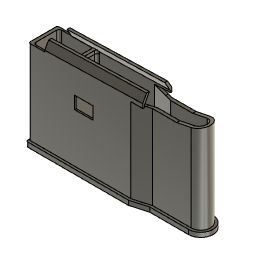
desert_tech_srs_magazine (Autodesk Fusion 360 design; units mm, degrees)
Autodesk Fusion 360 part; units mm, degrees
sketch "Sketch1" plane through (0, 0, 0) normal (0, 0, 1) x (1, 0, 0)
  line L0 (1.5, 0) -> (63.5, 0)
  line L1 (104.5, -3.8188) -> (104.5, 21.8188) construction
  line L2 (63.5, 18) -> (1.5, 18)
  line L3 (0, 16.25) -> (0, 1.5)
  line L4 (63.5, 18) -> (74, 15)
  line L5 (74, 15) -> (98, 15)
  line L6 (0, 9) -> (104.5, 9) construction
  arc A0 (104, 9) -> (98, 15) centre (98, 9) ccw
  line L7 (63.5, 0) -> (74, 3)
  line L8 (74, 3) -> (98, 3)
  arc A1 (98, 3) -> (104, 9) centre (98, 9) ccw
  line L9 (23.5, 15.5) -> (23.5, 10.6624)
  line L10 (25.5, 11.5003) -> (25.5, 15.5)
  line L11 (23.5, 2.5) -> (23.5, 7.3376)
  line L12 (25.5, 6.4997) -> (25.5, 2.5)
  arc A2 (100.0392, 12.4412) -> (98, 13) centre (98, 9) ccw
  line L13 (75.242, 13) -> (98, 13)
  line L14 (61.242, 17) -> (75.242, 13)
  line L15 (2, 15.5) -> (2, 2.5)
  line L16 (61.014, 1) -> (75.014, 5)
  line L17 (75.014, 5) -> (98, 5)
  arc A3 (98, 5) -> (100.0392, 12.4412) centre (98, 9) ccw
  line L18 (61.242, 17) -> (27, 17)
  line L19 (22, 17) -> (3.5, 17)
  line L20 (3.5, 1) -> (22, 1)
  line L21 (27, 1) -> (61.014, 1)
  line L22 (0, 1.5) -> (0, 0)
  line L23 (0, 0) -> (1.5, 0)
  line L24 (0, 16.25) -> (0, 18)
  line L25 (0, 18) -> (1.5, 18)
  line L26 (23.5, 10.6624) -> (23.5, 7.3376)
  line L27 (25.5, 11.5003) -> (25.5, 6.4997)
  arc A4 (27, 17) -> (25.5, 15.5) centre (27, 15.5) ccw
  arc A5 (25.5, 2.5) -> (27, 1) centre (27, 2.5) ccw
  arc A6 (23.5, 15.5) -> (22, 17) centre (22, 15.5) ccw
  arc A7 (22, 1) -> (23.5, 2.5) centre (22, 2.5) ccw
  arc A8 (3.5, 17) -> (2, 15.5) centre (3.5, 15.5) ccw
  arc A9 (2, 2.5) -> (3.5, 1) centre (3.5, 2.5) ccw
  point P0 (0, 18)
  dimension "d2" = 18
  dimension "d3" = 63.5
  dimension "d4" = 24
  dimension "d5" = 6.5
  dimension "d6" = 12
  dimension "d9" = 104.5
  dimension "d21" = 79
  dimension "d23" = 2
  dimension "d40" = 1
  dimension "d41" = 2
  dimension "d42" = 2
  dimension "d59" = 1.5
  dimension "d60" = 1.5
  dimension "d61" = 1.5
  dimension "d62" = 1.5
  dimension "d63" = 1.5
  dimension "d64" = 1.5
  dimension "d65" = 1
  constraint horizontal L0
  constraint vertical L1
  constraint horizontal L2
  constraint vertical L3
  constraint coincident L22.end L23.start
  constraint parallel L2 L5
  constraint midpoint L1 L6.end
  constraint coincident L6 A0.centre
  constraint tangent L5 A0
  constraint coincident L6 A0.start
  constraint symmetric L2.start L6 L0.end
  constraint symmetric L4.end L6 L7.end
  constraint symmetric L5.end L6 L8.end
  constraint symmetric L6 A0 A1
  constraint symmetric L6 A0.start A1.end
  constraint coincident L3 L6.start
  constraint coincident P0 L2
  constraint coincident P0 L3
  constraint coincident L22.end L3
  constraint coincident L22.end L0
  constraint symmetric L0 L2 L6
  constraint vertical L9
  constraint vertical L10
  constraint symmetric L6 L9.end L11.end
  constraint symmetric L6 L10.start L12.start
  constraint concentric A0 A2
  constraint parallel L5 L13
  constraint parallel L4 L14
  constraint parallel L2 L18
  constraint parallel L3 L15
  constraint parallel L0 L20
  constraint parallel L7 L16
  constraint parallel L8 L17
  constraint concentric A1 A3
  constraint tangent A2 A3
  constraint tangent A2 L13
  constraint tangent L17 A3
  constraint collinear L18 L19
  constraint collinear L20 L21
  constraint coincident P0 L24.end
  constraint parallel L12 L27
  constraint tangent L10 A4
  constraint tangent L18 A4
  constraint tangent L12 A5
  constraint tangent L21 A5
  constraint tangent L19 A6
  constraint tangent L9 A6
  constraint tangent L11 A7
  constraint tangent L20 A7
  constraint tangent L15 A8
  constraint tangent L19 A8
  constraint tangent L15 A9
  constraint tangent L20 A9
  constraint vertical L11
  measures "d2" distance of L22.end P0
  measures "d3" distance of L3 L2.start
  measures "d4" distance of L4.end L5.end
  measures "d5" distance of L1 L5.end
  measures "d6" diameter of A0
  measures "d9" distance of L1 L3
  measures "d21" distance of L1 L10
  measures "d23" distance of L9 L10
  measures "d40" distance of L2 L19
  measures "d41" distance of L5 L13
  measures "d42" distance of L3 L15
  measures "d59" radius of A4
  measures "d60" radius of A5
  measures "d61" radius of A6
  measures "d62" radius of A7
  measures "d63" radius of A8
  measures "d64" radius of A9
  measures "d65" distance of L0 L20
extrude "Extrude1" add sketch "Sketch1" along normal blind 55
sketch "Sketch2" plane through (0, 0, 0) normal (0, -1, 0) x (1, 0, 0)
  line L0 (0, 0) -> (63.5, 0)
  line L1 (63.5, 0) -> (63.5, 55)
  line L2 (63.5, 55) -> (0, 55)
  line L3 (28.5, 41) -> (40, 41)
  line L4 (40, 41) -> (40, 33.25)
  line L5 (40, 33.25) -> (28.5, 33.25)
  line L6 (28.5, 33.25) -> (28.5, 41)
  line L7 (0, 55) -> (0, 0)
  line L8 (0, 0) -> (0, 55)
  dimension "d25" = 7.75
  dimension "d26" = 11.5
  dimension "d28" = 14
  dimension "d36" = 28.5
  constraint horizontal L3
  constraint vertical L4
  constraint horizontal L5
  constraint vertical L6
  measures "d25" distance of L3 L5
  measures "d26" distance of L4 L6
  measures "d28" distance of L2 L3
  measures "d36" distance of L6 L8
extrude "Extrude2" cut sketch "Sketch2" against normal up to surface (1 mm away) contours L3 L4 L5 L6
sketch "Sketch4" plane through (0, 0, 0) normal (0, 1, 0) x (1, 0, 0)
  line L0 (0, -60) -> (70.8023, -62) construction
  line L1 (71, -55) -> (0, -55) construction
  line L2 (63.5, 0) -> (63.5, -55)
  line L3 (70.8023, -62) -> (71, -55)
  line L4 (63.5, -55) -> (74, -55)
  line L5 (0, -60) -> (0, -55) construction
  line L6 (10, -55) -> (10, -60.2825)
  line L7 (0, 0) -> (0, -55)
  line L8 (10, -60.2825) -> (70.8023, -62)
  line L9 (10, -55) -> (71, -55)
  point P0 (0, -55)
  dimension "d37" = 7
  dimension "d38" = 7.5
  dimension "d47" = 5
  dimension "d50" = 10
  constraint perpendicular L0 L3
  constraint coincident P0 L1.end
  constraint coincident L1.start L4
  constraint perpendicular L1 L5
  constraint coincident L1 L6.start
  constraint coincident L0 L6.end
  constraint perpendicular L1 L6
  measures "d37" distance of L0.end L1
  measures "d38" distance of L2.end L1.start
  measures "d47" distance of L1 L0.start
  measures "d50" distance of L6 L7
extrude "Extrude3" add sketch "Sketch4" along normal up to surface (18 mm away)
sketch "Sketch5" plane through (72.4958, 0, 2.0478) normal (0.999601, 0, 0.028236) x (0, 1, 0)
  line L0 (18, 52.9733) -> (18, 59.9761)
  line L1 (0, 59.9761) -> (0, 52.9733)
  line L2 (2.1429, 52.9733) -> (3.8531, 52.9733)
  line L3 (9, 63.92) -> (9, 36.6061) construction
  line L4 (1, 54.3074) -> (1, 52.9733)
  line L5 (0, 52.9733) -> (2.2125, 52.9733)
  line L6 (2.2125, 52.9733) -> (12.4801, 52.9733)
  line L7 (12.4801, 52.9733) -> (12.4801, 52.9731)
  line L8 (12.4801, 52.9731) -> (15.5375, 52.9731)
  line L9 (15.5375, 52.9731) -> (12.4801, 52.9731)
  line L10 (17.4429, 59.9761) -> (0, 59.9761)
  line L11 (0, 59.9761) -> (0, 52.9733)
  line L12 (1, 54.3074) -> (4.2, 59.9761)
  line L13 (0, 55.5873) -> (2.4775, 59.9761)
  line L14 (17, 54.3074) -> (13.8, 59.9761)
  line L15 (18, 55.5873) -> (15.5225, 59.9761)
  line L16 (17, 54.3074) -> (17, 52.9733)
  line L17 (18, 59.9761) -> (0, 59.9761)
  line L18 (0, 52.9733) -> (2.1429, 52.9733)
  line L19 (3.8531, 52.9733) -> (14.212, 52.9733)
  line L20 (14.212, 52.9733) -> (15.8571, 52.9733)
  line L21 (15.8571, 52.9733) -> (18, 52.9733)
  line L22 (18, 52.9733) -> (18, 59.9761)
  line L23 (18, 59.9761) -> (17.4429, 59.9761)
  dimension "d49" = 1.5
  dimension "d51" = 1
  dimension "d56" = 9.6
  constraint vertical L3
  constraint symmetric L0 L1 L3
  constraint coincident L10 L12.end
  constraint coincident L11 L13.start
  constraint coincident L10 L13.end
  constraint parallel L12 L13
  constraint parallel L1 L4
  constraint symmetric L3 L4.end L16.end
  constraint symmetric L3 L4.start L14.start
  constraint symmetric L3 L12.end L14.end
  constraint symmetric L3 L13.start L15.start
  constraint symmetric L3 L13.end L15.end
  constraint parallel L2 L6
  constraint parallel L1 L11
  constraint collinear L6 L19
  constraint horizontal L10
  constraint coincident L0.start L21.end
  constraint perpendicular L21 L22
  constraint coincident L15.start L22
  constraint collinear L10 L17
  constraint collinear L10 L23
  measures "d49" distance of L12 L13
  measures "d51" distance of L4 L11
  measures "d56" distance of L12.end L14.end
extrude "Extrude4" cut sketch "Sketch5" along normal up to surface contours L0 L10 L15 L17 L22 L23 | L2 L4 L5 L6 L8 L9 L10 L12 L14 L16 L17 L18 L19 L20 L21 | L1 L10 L11 L13 L17 end surface through (10, 0, 55) normal (-1, 0, 0) offset 0
sketch "Sketch8" plane through (0, 0, 0) normal (0, 0, -1) x (1, 0, 0)
  line L0 (61.242, -17) -> (27, -17)
  line L1 (25.5, -15.5) -> (25.5, -2.5)
  line L2 (27, -1) -> (61.014, -1)
  line L3 (61.014, -1) -> (75.014, -5)
  line L4 (75.014, -5) -> (98, -5)
  arc A0 (98, -13) -> (98, -5) centre (98, -9) ccw
  line L5 (98, -13) -> (75.242, -13)
  line L6 (75.242, -13) -> (61.242, -17)
  line L7 (2, -15.5) -> (2, -2.5)
  line L8 (23.5, -2.5) -> (23.5, -15.5)
  line L9 (0, 0) -> (0, -18)
  line L10 (0, -18) -> (63.5, -18)
  line L11 (63.5, -18) -> (74, -15)
  line L12 (74, -15) -> (98, -15)
  arc A1 (98, -15) -> (98, -3) centre (98, -9) ccw
  line L13 (98, -3) -> (74, -3)
  line L14 (74, -3) -> (63.5, 0)
  line L15 (63.5, 0) -> (0, 0)
  line L16 (0, -19.4407) -> (63.8085, -19.4407)
  line L17 (63.8085, -19.4407) -> (73.7522, -16.5997)
  line L18 (73.7522, -16.5997) -> (98, -16.5997)
  arc A2 (98, -16.5997) -> (98, -1.4003) centre (98, -9) ccw
  line L19 (98, -1.4003) -> (73.9484, -1.4003)
  line L20 (73.9484, -1.4003) -> (63.6749, 1.535)
  line L21 (63.6749, 1.535) -> (0, 1.535)
  line L22 (0, -18) -> (63.5, -18)
  line L23 (63.5, -18) -> (74, -15)
  line L24 (74, -15) -> (98, -15)
  arc A3 (98, -15) -> (98, -3) centre (98, -9) ccw
  line L25 (98, -3) -> (74, -3)
  line L26 (74, -3) -> (63.5, 0)
  line L27 (63.5, 0) -> (0, 0)
  line L28 (0, 0) -> (0, -18)
  line L29 (0, 0) -> (0, 1.535)
  line L30 (0, -18) -> (0, -19.4407)
  arc A4 (27, -1) -> (25.5, -2.5) centre (27, -2.5) ccw
  arc A5 (25.5, -15.5) -> (27, -17) centre (27, -15.5) ccw
  arc A6 (22, -17) -> (23.5, -15.5) centre (22, -15.5) ccw
  arc A7 (2, -15.5) -> (3.5, -17) centre (3.5, -15.5) ccw
  arc A8 (3.5, -1) -> (2, -2.5) centre (3.5, -2.5) ccw
  arc A9 (23.5, -2.5) -> (22, -1) centre (22, -2.5) ccw
  line L31 (22, -17) -> (3.5, -17)
  line L32 (3.5, -1) -> (22, -1)
  dimension "d53" = 0
  constraint coincident L9.start L15.end
  constraint perpendicular L21 L29
  constraint perpendicular L16 L30
  constraint parallel L10 L16
  constraint parallel L11 L17
  constraint parallel L12 L18
  constraint concentric A1 A2
  constraint parallel L13 L19
  constraint parallel L14 L20
  constraint parallel L15 L21
  constraint tangent A2 L19
  constraint tangent L18 A2
  measures "d53" distance of L10
extrude "Extrude5" add sketch "Sketch8" against normal blind 2.8 contours L10 L11 L12 A1 L13 L14 L15 L16 L17 L18 A2 L19 L20 L21 L22 L23 L24 A3 L25 L26 L27 L29 L30
fillet "Fillet1" radius 1 4 edges at (0, 0, 28.9) (0, 18, 28.9) (0, -1.535, 1.4) (0, 19.4407, 1.4)
extrude "Extrude6" add 3 faces at (24.8585, 15.9663, 53.6966) (24.8333, 13.4867, 53.6958) (24.1667, 9.1534, 53.6771) along direction (-0.028236, 0, 0.999601) blind 2
sketch "Sketch9" plane through (0, 3, 0) normal (0, -1, 0) x (1, 0, 0)
  line L0 (74, 2.8) -> (98, 2.8)
  line L1 (98, 2.8) -> (98, 55)
  line L2 (98, 55) -> (74, 55)
  line L3 (74, 55) -> (74, 2.8)
  line L4 (89, 55) -> (104, 58)
  line L5 (104, 58) -> (104, 55)
  line L6 (104, 55) -> (89, 55)
  dimension "d81" = 15
  dimension "d82" = 3
  constraint coincident L2 L4.start
  constraint perpendicular L2 L5
  constraint perpendicular L5 L6
  measures "d81" distance of L4.start L5.end
  measures "d82" distance of L4.end L5.end
extrude "Extrude7" add sketch "Sketch9" against normal up to surface (12 mm away) contours L2 L4 L5 L6
extrude "Extrude11" cut 3 faces at (102.8212, 13.8212, 55) (95, 7.6667, 55) (102.8212, 4.1788, 55) along direction (0, 0, -1) up to surface end surface through (89, 3, 55) normal (-0.196116, 0, 0.980581) offset 0
